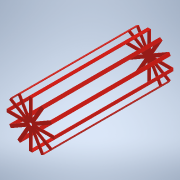
# Autodesk Inventor part: Rubber Band
Saved by Autodesk Inventor 2022 (Build 260153070, 153G)
## iProperties
Created: 2021-04-03
Part Number: Rubber Band
Material: Generic
Document SubType Name: Modeling
Designer: arybo
Density: 1 g/cm^3
Appearance: Default
Author: arybo
Autodesk Inventor part; units mm, degrees
ref_plane "YZ Plane" through (0, 0, 0) normal (1, 0, 0) x (0, 1, 0)
ref_plane "XZ Plane" through (0, 0, 0) normal (0, 1, 0) x (-1, 0, 0)
ref_plane "XY Plane" through (0, 0, 0) normal (0, 0, 1) x (1, 0, 0)
sketch "Sketch1" plane through (0, 0, 0) normal (0, 0, 1) x (1, 0, 0)
  line L0 (0, 0) -> (72.39, 0)
  line L1 (72.39, 0) -> (72.39, -4.7625)
  line L2 (0, 0) -> (0, -4.7625)
  line L3 (0, -4.7625) -> (72.39, -4.7625)
  circle A0 centre (36.195, -2.3813) radius 2.2098
  dimension "d0" = 72.39
  dimension "d1" = 4.7625
  dimension "d2" = 4.7625
  dimension "d3" = 4.4196
  constraints: 8 end point, 1 centre point, 1 horizontal, 1 perpendicular, 1 vertical
  measures "d0" distance of L0.start L0.end
  measures "d1" distance of L0.end L1.end
  measures "d2" distance of L0.start L2.end
  measures "d3" diameter of A0
extrude "Extrusion1" add sketch "Sketch1" along normal blind 0.7937
sketch "Sketch2" plane through (0, -4.7625, 0) normal (-1, 0, 0) x (0, 0, 1)
  line L0 (0, 0) -> (0, 4.7625) projected
  line L1 (0, 4.7625) -> (-179.451, 4.7625)
  line L2 (-179.451, 4.7625) -> (-179.451, 0)
  line L3 (-179.451, 0) -> (0, 0)
  dimension "d6" = 179.451
  constraints: 6 end point, 2 perpendicular, 1 horizontal
  measures "d6" distance of L0.end L1.end
extrude "Extrusion2" add sketch "Sketch2" against normal blind 0.7937
sketch "Sketch3" plane through (0, -4.7625, -179.451) normal (0, 0, -1) x (-1, 0, 0)
  line L0 (0, 4.7625) -> (0, 0) projected
  line L1 (-72.39, 0) -> (-72.39, 4.7625) projected
  line L2 (0, 4.7625) -> (-72.39, 4.7625)
  line L3 (-72.39, 4.7625) -> (-72.39, 0)
  line L4 (-72.39, 0) -> (0, 0)
  line L5 (0, 0) -> (0, 4.7625)
  constraints: 8 end point, 3 perpendicular, 1 collinear
extrude "Extrusion3" add sketch "Sketch3" along normal blind 0.7937
sketch "Sketch4" plane through (72.39, -4.7625, 0) normal (1, 0, 0) x (0, 0, -1)
  line L0 (0, 0) -> (0, 4.7625) projected
  line L1 (179.451, 4.7625) -> (0, 4.7625) projected
  line L2 (0, 4.7625) -> (179.451, 4.7625)
  line L3 (0, 0) -> (179.451, 0) projected
  line L4 (179.451, 4.7625) -> (179.451, 0)
  line L5 (179.451, 0) -> (0, 0)
  line L6 (0, 0) -> (0, 4.7625)
  constraints: 8 end point, 3 perpendicular, 1 collinear
extrude "Extrusion4" add sketch "Sketch4" against normal blind 0.7937
pattern_circular "Circular Pattern1" count 12 over 360 about axis through (36.195, -2.3813, 0) along (0, 0, 1) of "Extrusion3", "Extrusion2", "Extrusion1", "Extrusion4"
body "Solid1"
